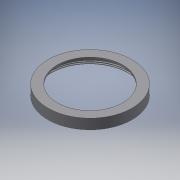
# Autodesk Inventor part: Bauteil5
Saved by Autodesk Inventor 2016 SP2 (Build 200236200, 236)
## iProperties
Created: 2018-09-27
Part Number: Bauteil5
Material: Generisch
Document SubType Name: Modeling
Designer: Nils
Density: 1 g/cm^3
Appearance: Vorgabe
Author: Nils
Autodesk Inventor part; units mm, degrees
ref_plane "YZ Plane" through (0, 0, 0) normal (1, 0, 0) x (0, 1, 0)
ref_plane "XZ Plane" through (0, 0, 0) normal (0, 1, 0) x (-1, 0, 0)
ref_plane "XY Plane" through (0, 0, 0) normal (0, 0, 1) x (1, 0, 0)
sketch "Skizze2" plane through (0, 0, 0) normal (0, 1, 0) x (-1, 0, 0)
  line L0 (50, 0) -> (47.7, 0)
  line L1 (47.7, 0) -> (47.7, 3)
  line L2 (47.7, 3) -> (47, 3)
  line L3 (47, 3) -> (47, 10)
  line L4 (47, 10) -> (39, 10)
  line L5 (39, 10) -> (39, 12)
  line L6 (39, 12) -> (50, 12)
  line L7 (50, 12) -> (50, 0)
  line L8 (0, -2.4) -> (0, 14.4) projected
  point P0 (0, 0)
  dimension "d0" = 2.3
  dimension "d1" = 3
  dimension "d3" = 7
  dimension "d4" = 8
  dimension "d5" = 2
  dimension "d6" = 50
  dimension "d7" = 0
  dimension "d29" = 3
  constraints: 16 end point, 7 perpendicular, 1 horizontal
  measures "d0" distance of L0.start L0.end
  measures "d1" distance of L0.end L1.end
  measures "d3" distance of L2.end L3.end
  measures "d4" distance of L3.end L4.end
  measures "d5" distance of L4.end L5.end
  measures "d6" distance from line of point (0, 0) L7
  measures "d7" distance from line of point (0, 0) L0
  measures "d29" distance between parallel lines of L7 L3
revolve "Umdrehung1" add sketch "Skizze2" angle 360 about axis through (0, 0, -10) along (0, 0, 1)
thread "Gewinde2" size "M95x2" class "6H" standard "ANSI Metric M Profile" full length
sketch "Skizze6" plane through (0, 0, 0) normal (1, 0, 0) x (0, 1, 0)
  line L0 (47.7, 0) -> (47.7, 3)
  line L1 (47.7, 3) -> (46.3948, 3)
  line L2 (46.3948, 3) -> (46.3948, 0)
  line L3 (46.3948, 0) -> (47.7, 0)
  line L4 (0, -5.0391) -> (0, 14.8398) projected
  constraints: 8 end point
revolve "Umdrehung3" add sketch "Skizze6" angle 360 about axis through (0, 0, 0) along (0, 0, 1) separate body
sketch "Skizze5" plane through (0, 47.7, 0) normal (-1, 0, 0) x (0, 0, 1)
  line L0 (-1.1849, -0.1069) -> (-1.0001, -0.1069) construction
  line L1 (0.1847, -1.1986) -> (-0.0001, -1.5188) construction
  line L2 (-2.0001, -1.5188) -> (-2.185, -1.1986) construction
  line L3 (-0.8153, -0.1069) -> (-1.0001, 0.2133) construction
  line L4 (-1.0001, 0.2133) -> (-1.1849, -0.1069) construction
  line L5 (-2.0001, -1.5188) -> (-1.8153, -1.1986) construction
  line L6 (-0.8153, -0.1069) -> (-0.1849, -1.1986)
  line L7 (-2.185, -1.1986) -> (-1.8153, -1.1986) construction
  arc A0 (-2.185, -1.1986) -> (-2.0001, -1.3053) centre (-2.0001, -1.0919) ccw construction
  line L8 (0.1847, -1.1986) -> (-0.1849, -1.1986) construction
  line L9 (-2.0001, -1.5188) -> (-2.0001, -1.1986) construction
  line L10 (-0.0001, -1.5188) -> (-0.0001, -1.1986) construction
  line L11 (-1.0001, 0.2133) -> (-1.0001, -0.0002) construction
  line L12 (-2.0001, -1.3053) -> (-0.0001, -1.3053)
  arc A1 (-2.0001, -1.3053) -> (-1.8153, -1.1986) centre (-2.0001, -1.0919) ccw
  line L13 (-0.1849, -1.1986) -> (-0.0001, -1.5188) construction
  line L14 (-1.8153, -1.1986) -> (-1.1849, -0.1069)
  line L15 (-0.0001, -0.0002) -> (-0.0001, 0.0177)
  line L16 (-0.0001, 0.0177) -> (-0.0001, -0.0002)
  line L17 (-0.0001, -0.0002) -> (0.0334, -0.0002)
  arc A2 (-0.1849, -1.1986) -> (-0.0001, -1.3053) centre (-0.0001, -1.0919) ccw
  arc A3 (-0.0001, -1.3053) -> (0.1847, -1.1986) centre (-0.0001, -1.0919) ccw construction
  arc A4 (-1.0001, -0.0002) -> (-1.1849, -0.1069) centre (-1.0001, -0.2136) ccw
  arc A5 (-0.8153, -0.1069) -> (-1.0001, -0.0002) centre (-1.0001, -0.2136) ccw
  line L18 (-1.0001, -0.0002) -> (-1.0001, -0.1069) construction
  line L19 (-1.0001, -0.1069) -> (-0.8153, -0.1069) construction
  dimension "d32" = 60
  dimension "d33" = 0.3202
  dimension "d34" = 0.3202
  dimension "Skizze5_ThreadOffset" = 0
  dimension "Skizze5_MajorRadius" = 1.3052
  dimension "d37" = 2
  dimension "Skizze5_MinorRadius" = 0
  constraints: 40 end point, 12 point on circle, 10 parallel, 8 tangent, 6 centre point, 6 collinear, 2 midpoint, 2 point on line, 1 horizontal, 1 perpendicular, 3 other
  measures "d32" angle of L6 L14
  measures "d33" distance of L3.end L0.end
  measures "d34" distance of L1.end L10.end
  measures "Skizze5_ThreadOffset" distance between parallel lines of L15 L10
  measures "Skizze5_MajorRadius" distance from line of L12 L15.start
  measures "d37" distance from line of L1.end L9
  measures "Skizze5_MinorRadius" distance edge to line of A5 L17
coil "Spirale2" sketch "Skizze5" operation cut axis through (0, 0, 0) along (0, 0, 1) pitch 2.002 turns 3.496503 hand right bodies 2
equation "\"d32\" = d39"
equation "\"d33\" = 0.160083 * Skizze5_Pitch"
equation "\"d34\" = 0.160083 * Skizze5_Pitch"
equation "\"d37\" = Skizze5_Pitch"
equation "\"d18\" = 60deg"
equation "\"Skizze3_Pitch\" = 2"
equation "\"d39\" = 60deg"
equation "\"Skizze5_Pitch\" = 2"
